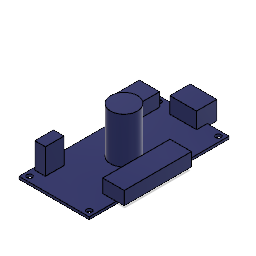
gimbal_base_intel (Autodesk Fusion 360 archive; units mm, degrees)
design "sensorimotor_board"
Autodesk Fusion 360 part; units mm, degrees
sketch "Sketch1" plane through (0, 0, 0) normal (0, 1, 0) x (1, 0, 0)
  line L0 (0, 0) -> (26.2, 0)
  line L1 (26.2, 0) -> (26.2, -52)
  line L2 (26.2, -52) -> (0, -52)
  line L3 (0, -52) -> (0, 0)
  circle A0 centre (2, -2) radius 1
  circle A1 centre (24.2, -2) radius 1
  line L4 (0, -26) -> (26.2, -26)
  circle A2 centre (2, -50) radius 1
  circle A3 centre (24.2, -50) radius 1
  dimension "d1" = 52
  dimension "d2" = 26.2
  dimension "d3" = 2
  dimension "d4" = 2
  dimension "d5" = 2
  dimension "d6" = 2
  dimension "d7" = 2
  dimension "d8" = 2
  constraint horizontal L0
  constraint vertical L1
  constraint horizontal L2
  constraint vertical L3
  constraint coincident L0.start L3.end
  constraint midpoint L3 L4.start
  constraint midpoint L1 L4.end
  constraint symmetric A0 L4 A2
  constraint symmetric A1 L4 A3
  measures "d1" distance of L0.start L2.end
  measures "d2" distance of L0.start L0.end
  measures "d3" diameter of A0
  measures "d4" distance of L0 A0.centre
  measures "d5" distance of L3 A0.centre
  measures "d6" diameter of A1
  measures "d7" distance of L0 A1.centre
  measures "d8" distance of L1 A1.centre
extrude "Extrude1" add sketch "Sketch1" along normal blind 1
sketch "Sketch2" plane through (0, 1, 0) normal (0, 1, 0) x (-1, 0, 0)
  circle A0 centre (-2, 2) radius 1
  circle A1 centre (-24.2, 2) radius 1
  circle A2 centre (-2, 50) radius 1
  circle A3 centre (-24.2, 50) radius 1
  line L0 (0, 52) -> (-26.2, 52)
  line L1 (-26.2, 52) -> (-26.2, 0)
  line L2 (-26.2, 0) -> (0, 0)
  line L3 (0, 0) -> (0, 52)
  line L4 (-1, 47.0961) -> (-5, 47.0961)
  line L5 (-5, 47.0961) -> (-5, 40.0961)
  line L6 (-5, 40.0961) -> (-1, 40.0961)
  line L7 (-1, 40.0961) -> (-1, 47.0961)
  line L8 (-21.2, 42) -> (-29.2, 42)
  line L9 (-29.2, 42) -> (-29.2, 17)
  line L10 (-29.2, 17) -> (-21.2, 17)
  line L11 (-21.2, 17) -> (-21.2, 42)
  line L12 (0, 3.6) -> (-4, 3.6)
  line L13 (-4, 3.6) -> (-4, 13.6)
  line L14 (-4, 13.6) -> (0, 13.6)
  line L15 (0, 13.6) -> (0, 3.6)
  line L16 (0, 3.6) -> (3.6, 3.6)
  line L17 (3.6, 3.6) -> (3.6, 13.6)
  line L18 (3.6, 13.6) -> (0, 13.6)
  line L19 (0, 13.6) -> (0, 3.6)
  dimension "d11" = 4
  dimension "d12" = 7
  dimension "d15" = 3
  dimension "d16" = 25
  dimension "d17" = 8
  dimension "d18" = 10
  dimension "d29" = 4
  dimension "d30" = 10
  dimension "d31" = 3.6
  dimension "d32" = 3.6
  constraint horizontal L4
  constraint vertical L5
  constraint horizontal L6
  constraint vertical L7
  constraint horizontal L8
  constraint vertical L9
  constraint horizontal L10
  constraint vertical L11
  constraint horizontal L12
  constraint vertical L13
  constraint horizontal L14
  constraint vertical L15
  constraint coincident L3 L12.start
  constraint horizontal L16
  constraint vertical L17
  constraint horizontal L18
  constraint vertical L19
  measures "d11" distance of L4.start L4.end
  measures "d12" distance of L4.start L6.end
  measures "d15" distance of L1 L9
  measures "d16" distance of L8.end L9.end
  measures "d17" distance of L9.end L10.end
  measures "d18" distance of L0 L8
  measures "d29" distance of L12.start L12.end
  measures "d30" distance of L12.start L14.end
  measures "d31" distance of L2 L12
  measures "d32" distance of L14.end L17.end
extrude "Extrude2" add sketch "Sketch2" along normal blind 9.5 contours L4 L5 L6 L7
extrude "Extrude3" add sketch "Sketch2" along normal blind 5 contours L1 L8 L10 L11 | L1 L8 L9 L10
sketch "Sketch3" plane through (0, 0, 0) normal (0, -1, 0) x (1, 0, 0)
  circle A0 centre (2, 2) radius 1
  circle A1 centre (24.2, 2) radius 1
  circle A2 centre (2, 50) radius 1
  circle A3 centre (24.2, 50) radius 1
  line L0 (26.2, 52) -> (0, 52)
  line L1 (0, 52) -> (0, 0)
  line L2 (0, 0) -> (26.2, 0)
  line L3 (26.2, 0) -> (26.2, 52)
  circle A4 centre (13.1, 26) radius 5
  line L4 (18.1, 0) -> (8.1, 0)
  line L5 (8.1, 0) -> (8.1, 4)
  line L6 (8.1, 4) -> (18.1, 4)
  line L7 (18.1, 4) -> (18.1, 0)
  line L8 (8.1, 0) -> (0, 0)
  line L9 (18.1, 0) -> (26.2, 0)
  line L10 (8.1, 0) -> (18.1, 0)
  line L11 (18.1, 0) -> (18.1, -3.6)
  line L12 (18.1, -3.6) -> (8.1, -3.6)
  line L13 (8.1, -3.6) -> (8.1, 0)
  point P0 (13.1, 26)
  dimension "d21" = 10
  dimension "d24" = 10
  dimension "d25" = 4
  dimension "d26" = 3.6
  constraint coincident P0 A4.centre
  constraint horizontal L4
  constraint vertical L5
  constraint horizontal L6
  constraint vertical L7
  constraint coincident L2 L4.start
  constraint coincident L1.end L2.start
  constraint coincident L2.end L3.start
  constraint equal L8 L9
  constraint horizontal L10
  constraint vertical L11
  constraint horizontal L12
  constraint vertical L13
  measures "d21" diameter of A4
  measures "d24" distance of L5.end L6.end
  measures "d25" distance of L4.end L5.end
  measures "d26" distance of L4.end L12.end
extrude "Extrude4" add sketch "Sketch3" against normal blind 18 contours A4
extrude "Extrude5" add sketch "Sketch3" against normal blind 7 contours L2 L4 L10 L11 L12 L13 | L2 L4 L5 L6 L7 L10
extrude "Extrude6" add sketch "Sketch2" along normal blind 5 contours L3 L15 L16 L17 L18 L19 | L3 L12 L13 L14 L15 L19
